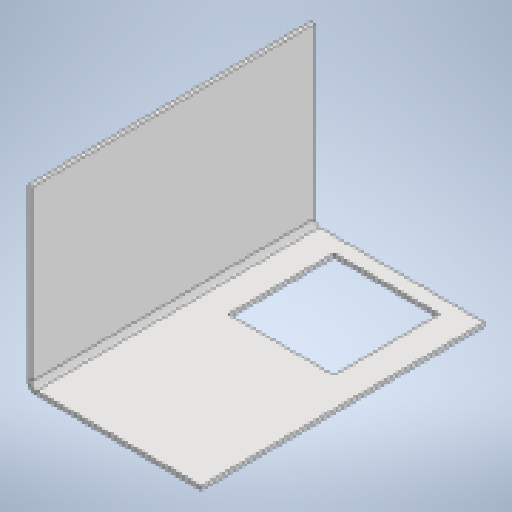
# Autodesk Inventor part: SLM 1652 FDS Central tube wall
Saved by Autodesk Inventor 2025.4 (Build 294407000, 407)
## iProperties
Created: 2025-06-24
Part Number: SLM 1652 FDS Central tube wall
Material: Stainless Steel
Document SubType Name: Sheet Metal
Designer: admin
Mass: 345.577 g
Surface Area: 451.507 cm^2
Volume: 43.1971 cm^3
Density: 8 g/cm^3
Flat Pattern Width: 18.2202 cm
Flat Pattern Length: 15 cm
Flat Pattern Area: 273.303 cm^2
Sheet Metal Rule: AISI304 2mm Die16
Sheet Metal Width: 182,202 mm
Sheet Metal Length: 150,000 mm
Sheet Metal Area: 27330,299 mm^2
Appearance: Default
Author: user
Autodesk Inventor part; units mm, degrees
ref_plane "YZ Plane" through (0, 0, 0) normal (1, 0, 0) x (0, 1, 0)
ref_plane "XZ Plane" through (0, 0, 0) normal (0, 1, 0) x (-1, 0, 0)
ref_plane "XY Plane" through (0, 0, 0) normal (0, 0, 1) x (1, 0, 0)
sketch "Sketch1" plane through (0, 0, 0) normal (0, 0, 1) x (1, 0, 0)
  line L0 (-46, -75) -> (46, -75)
  line L1 (46, -75) -> (46, 75)
  line L2 (46, 75) -> (-46, 75)
  line L3 (-46, 75) -> (-46, -75)
  line L4 (-46, -75) -> (46, 75) construction
  line L5 (46, -75) -> (-46, 75) construction
  point P0 (0, 0)
  dimension "d154" = 92
  dimension "d155" = 150
  measures "d154" distance of L1.end L2.end
  measures "d155" distance of L0.end L1.end
extrude "Plate5" add sketch "Sketch1" along normal blind 2
sketch "Sketch7" plane through (-44, -75, 0) normal (-1, 0, 0) x (0, -1, 0)
  line L0 (-150, 0) -> (0, 0)
  line L1 (0, 0) -> (0, 94)
  line L2 (0, 94) -> (-150, 94)
  line L3 (-150, 94) -> (-150, 0)
  constraints: 6 end point, 1 horizontal, 1 perpendicular, 1 vertical
edge flange "Flange3" height 94 angle 90 thickness 2 bend radius 2.75 thickness toward (-1, 0, 0) relief round relief width 2 relief depth 1 edges at (-46, 0, 2) wall of the first edge with corners at (-44, 75, 0) (-44, -75, 0) (-44, -75, 94) (-44, 75, 94)
bend "Bend3"
corner "Corner3"
sketch "Sketch8" plane through (0, 0, 2) normal (0, 0, 1) x (1, 0, 0)
  line L0 (46, 75) -> (46, -75) projected
  line L1 (-41.25, 75) -> (46, 75) projected
  line L2 (30.375, 67) -> (-25.625, 67)
  line L3 (-25.625, 67) -> (-25.625, 11)
  line L4 (-25.625, 11) -> (30.375, 11)
  line L5 (30.375, 11) -> (30.375, 67)
  line L6 (30.375, 67) -> (-25.625, 11) construction
  line L7 (-25.625, 67) -> (30.375, 11) construction
  point P0 (0, 0)
  point P1 (2.375, 39)
  point P2 (2.375, 75)
  dimension "d167" = 56
  dimension "d168" = 56
  dimension "d169" = 8
  constraints: 12 end point, 3 midpoint, 2 parallel, 1 horizontal, 1 perpendicular, 1 vertical alignment
  measures "d167" distance of L4.end L3.end
  measures "d168" distance of L3.end L2.end
  measures "d169" distance between parallel lines of L1 L2
extrude "Cut1" cut sketch "Sketch8" against normal blind 2
sketch "Sketch9" plane through (-46, -75, 94) normal (-1, 0, 0) x (0, 0, 1)
  line L0 (-29.375, 94.75) -> (-59.875, 94.75)
  line L1 (-59.875, 94.75) -> (-59.875, 125.25)
  line L2 (-59.875, 125.25) -> (-29.375, 125.25)
  line L3 (-29.375, 125.25) -> (-29.375, 94.75)
  line L4 (-29.375, 94.75) -> (-59.875, 125.25) construction
  line L5 (-59.875, 94.75) -> (-29.375, 125.25) construction
  circle A0 centre (-19.625, 85) radius 2.5
  circle A1 centre (-69.625, 85) radius 2.5
  circle A2 centre (-69.625, 135) radius 2.5
  circle A3 centre (-19.625, 135) radius 2.5
  circle A4 centre (-44.625, 110) radius 35.3553 construction
  line L6 (-59.875, 94.75) -> (-69.625, 85) construction
  line L7 (-17.125, 82.5) -> (-72.125, 82.5) construction
  line L8 (-72.125, 82.5) -> (-72.125, 137.5) construction
  line L9 (-72.125, 137.5) -> (-17.125, 137.5) construction
  line L10 (-17.125, 137.5) -> (-17.125, 82.5) construction
  line L11 (-17.125, 82.5) -> (-72.125, 137.5) construction
  line L12 (-72.125, 82.5) -> (-17.125, 137.5) construction
  line L13 (-89.25, 150) -> (0, 150) projected
  line L14 (-44.625, 150) -> (-44.625, 110) construction
  circle A5 centre (-69.625, 135) radius 13.7886 construction
  line L15 (-19.625, 85) -> (-69.625, 85) construction
  line L16 (-69.625, 85) -> (-69.625, 135) construction
  line L17 (-69.625, 135) -> (-19.625, 135) construction
  line L18 (-19.625, 135) -> (-19.625, 85) construction
  line L19 (-19.625, 85) -> (-69.625, 135) construction
  line L20 (-69.625, 85) -> (-19.625, 135) construction
  point P0 (-94, 75)
  point P1 (-104.8197, 150.8767)
  point P2 (-104.8197, 150.8767)
  dimension "d181" = 27.5772
  dimension "d174" = 30.5
  dimension "d175" = 30.5
  dimension "d176" = 5
  dimension "d179" = 40
  dimension "d180" = 55
  dimension "d184" = 50
  constraints: 40 end point, 7 midpoint, 6 parallel, 5 centre point, 5 point on line, 4 point on circle, 3 equal radius, 3 horizontal, 3 perpendicular, 2 coincident, 1 tangent, 1 vertical, 3 other
  measures "d174" distance of L3.end L1.start
  measures "d175" distance of L1.start L1.end
  measures "d176" diameter of A0
  measures "d179" distance from line of L14.end L13
  measures "d180" distance of L7.end L8.end
  measures "d184" distance of L17.end L15.start
extrude "Cut2" cut sketch "Sketch9" against normal blind 2
body "Solid3"
